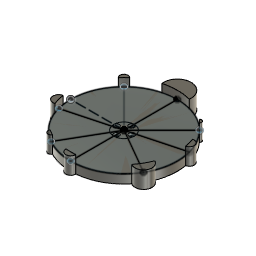
Baseplate_v3 (Autodesk Fusion 360 design; units mm, degrees)
Autodesk Fusion 360 part; units mm, degrees
note: some values were not read from the file. Set by a fixed rule: which face or edge a step refers to.
sketch "Sketch1" plane through (0, 0, 0) normal (0, 0, 1) x (1, 0, 0) in component "Component"
  circle A0 centre (0, 0) radius 60
  circle A1 centre (0, 0) radius 11.5
  dimension "d1" = 120
  dimension "d2" = 23
  constraint coincident A0.centre A1.centre
  measures "d1" diameter of A0
  measures "d2" diameter of A1
extrude "Extrude1" add sketch "Sketch1" along normal blind 5 makes body 1 in component "Component"
sketch "Sketch1 (2)" plane through (0, 0, 5) normal (0, 0, 1) x (-1, 0, 0) in component "Component'"
  circle A0 centre (0, 0) radius 11.5
  circle A1 centre (0, 0) radius 60
  circle A2 centre (0, 0) radius 11.5
  constraint concentric A0 A2
extrude "Extrude1'" add sketch "Sketch1 (2)" along normal blind 2 separate body contours A0 A2 makes body 2 in component "Component'"
move_face "MoveFace1" to x (1, 0, 0) y (0, 1, 0) z (0, 0, 1) at (0, 0, -5) 1 faces at (-11.4857, 0.5732, 6.3333) on bodies 2 in component "Component'"
sketch "Sketch2" plane through (0, 0, 7) normal (0, 0, 1) x (-1, 0, 0) in component "Component'"
  circle A0 centre (0, 0) radius 11.5
sketch "Sketch1 (3)" plane through (0, 0, 7) normal (0, 0, 1) x (-1, 0, 0) in component "Component''"
  circle A0 centre (0, 0) radius 11.5
  circle A1 centre (8.5, 0) radius 1.5
  circle A2 centre (0, -8.5) radius 1.5
  circle A3 centre (-8.5, 0) radius 1.5
  circle A4 centre (0, 8.5) radius 1.5
  dimension "d7" = 23
  dimension "d8" = 3
  dimension "d9" = 3
  dimension "d10" = 3
  dimension "d11" = 3
  measures "d7" diameter of A0
  measures "d8" diameter of A1
  measures "d9" diameter of A2
  measures "d10" diameter of A3
  measures "d11" diameter of A4
extrude "Extrude2" cut sketch "Sketch1 (3)" against normal blind 4.5 contours A1 | A2 | A3 | A4 bodies 2 in component "Component'"
extrude "Extrude2'" add 1 faces at (43.5671, -3.5522, 5) along direction (0, 0, 1) blind 5 on bodies 1 bodies 1 in component "Component"
sketch "Sketch1 (4)" plane through (0, 0, 7) normal (0, 0, 1) x (-1, 0, 0) in component "Component'''"
  circle A0 centre (-8.5, 0) radius 2.5
  circle A1 centre (0, 8.5) radius 2.5
  circle A2 centre (8.5, 0) radius 2.5
  circle A3 centre (0, -8.5) radius 2.5
  dimension "d16" = 5
  dimension "d17" = 5
  dimension "d18" = 5
  dimension "d19" = 5
  measures "d16" diameter of A0
  measures "d17" diameter of A1
  measures "d18" diameter of A2
  measures "d19" diameter of A3
extrude "Extrude3" add sketch "Sketch2" along normal blind 3 bodies 2 in component "Component'"
extrude "Extrude4" cut sketch "Sketch1 (4)" along normal blind 7.5 bodies 2 in component "Component'"
hole "Hole1" at (-8.5, 0, 10) direction (0, 0, -1) diameter 6 depth 3 tip angle 180 bodies 2 in component "Component'"
hole "Hole2" at (0, -8.5, 10) direction (0, 0, -1) diameter 6 depth 3 tip angle 180 bodies 2 in component "Component'"
hole "Hole3" at (8.5, 0, 10) direction (0, 0, -1) diameter 6 depth 3 tip angle 180 bodies 2 in component "Component'"
hole "Hole4" at (0, 8.5, 10) direction (0, 0, -1) diameter 6 depth 3 tip angle 180 bodies 2 in component "Component'"
sketch "Sketch1 (5)" plane through (0, 0, 10) normal (0, 0, 1) x (-1, 0, 0) in component "poles"
  circle A0 centre (0, 0) radius 11.5
  circle A1 centre (0, 0) radius 60
  circle A2 centre (0, 0) radius 60
  line L0 (0, 0) -> (57.9555, 15.5291)
  line L1 (0, 0) -> (60, 0) construction
  line L2 (0, 0) -> (30, 51.9615)
  line L3 (0, 0) -> (60, 0) construction
  line L4 (0, 0) -> (0, 60)
  line L5 (0, 0) -> (-51.9615, 30)
  line L6 (0, 0) -> (-57.9555, -15.5291)
  line L7 (0, 0) -> (60, 0) construction
  line L8 (0, 0) -> (42.4264, -42.4264)
  line L9 (0, 0) -> (60, 0) construction
  line L10 (0, 0) -> (0, -60)
  line L11 (0, 0) -> (-42.4264, -42.4264)
  circle A3 centre (42.4264, -42.4264) radius 2.5
  circle A4 centre (42.4264, -42.4264) radius 2.5
  circle A5 centre (0, -60) radius 2.5
  circle A6 centre (-42.4264, -42.4264) radius 2.5
  circle A7 centre (60, 0) radius 2.5
  circle A8 centre (57.9555, 15.5291) radius 2.5
  circle A9 centre (30, 51.9615) radius 2.5
  circle A10 centre (0, 60) radius 2.5
  circle A11 centre (-51.9615, 30) radius 2.5
  dimension "d36" = 15
  dimension "d37" = 60
  dimension "d38" = 60
  dimension "d39" = 165
  dimension "d40" = 60
  dimension "d41" = 45
  dimension "d42" = 135
  dimension "d43" = 5
  dimension "d44" = 5
  dimension "d45" = 5
  dimension "d46" = 5
  dimension "d47" = 5
  dimension "d48" = 5
  dimension "d49" = 5
  dimension "d50" = 5
  dimension "d51" = 5
  constraint concentric A0 A2
  constraint horizontal L1
  constraint coincident A0.centre A1.centre
  constraint horizontal L3
  constraint vertical L4
  constraint coincident A2 L5.end
  constraint perpendicular L2 L5
  constraint horizontal L7
  constraint horizontal L9
  constraint coincident A2 L10.end
  constraint perpendicular L7 L10
  constraint coincident L8.end A3.centre
  constraint coincident L10.end A5.centre
  constraint coincident L11.end A6.centre
  constraint coincident L1.end L3.end
  constraint coincident L0.end A8.centre
  constraint coincident L2.end A9.centre
  constraint coincident L4.end A10.centre
  constraint coincident L5.end A11.centre
  measures "d36" angle of L0 L1
  measures "d37" angle of L2 L3
  measures "d38" distance of A0.centre L5.end
  measures "d39" angle of L6 L7
  measures "d40" distance of A0.centre L6.end
  measures "d41" angle of L8 L9
  measures "d42" angle of L10 L11
  measures "d43" diameter of A3
  measures "d44" diameter of A4
  measures "d45" diameter of A5
  measures "d46" diameter of A6
  measures "d47" diameter of A7
  measures "d48" diameter of A8
  measures "d49" diameter of A9
  measures "d50" diameter of A10
  measures "d51" diameter of A11
extrude "Extrude1''" add sketch "Sketch1 (5)" along normal blind 9 separate body contours A1 A2 A8 | A1 A2 A3 A4 | A1 A2 A9 | A1 A2 A7 | A1 A2 A5 | A1 A2 A10 | A1 A2 A11 | A1 A2 A6 picked at (60.7968, -0.5156) makes body 3 at (2.0546, 61.4243, 13) makes body 4 at (-2.4929, -60.1889, 16) makes body 5 at (-59.9493, -17.0374, 13) makes body 6 at (40.7077, 44.2419, 16) makes body 7 at (-44.0157, 44.3562, 13) makes body 8 at (-32.4952, -51.8063, 13) makes body 9 at (-60.1889, -2.4929, 13) makes body 10 at (53.8468, -31.6419, 16) in component "poles"
extrude "Extrude2''" add 8 faces at (0, -60.8295, 10) (-30.4147, -52.6799, 10) (-58.7568, -15.7438, 10) (-60.8295, 0, 10) (-43.0129, 43.0129, 10) (43.0129, 43.0129, 10) (52.6799, -30.4147, 10) (0, 60.8295, 10) along direction (0, 0, -1) blind 10 on bodies 3 4 5 6 7 8 9 10 bodies 4 3 5 6 7 8 9 10 in component "poles"
move_body "Move1" bodies 9 to x (-0.965926, -0.258819, 0) y (0.258819, -0.965926, 0) z (0, 0, 1) at (-0.0081, 0.0136, 0) in component "poles"
extrude "Extrude3'" add 2 faces at (0, 60.8295, 19) (-30.4147, -52.6799, 19) along direction (0, 0, -1) blind 4 on bodies 3 8 bodies 3 8 in component "poles"
extrude "Extrude4'" cut 2 faces at (0, -60.8295, 19) (43.0129, 43.0129, 19) along direction (0, 0, 1) blind 6.5 on bodies 4 6 bodies 4 6 in component "poles"
extrude "Extrude5" add 2 faces at (58.7487, 15.7575, 19) (-43.0129, 43.0129, 19) along direction (0, 0, -1) blind 1 on bodies 7 9 bodies 9 7 in component "poles"
move_face "OffsetFaces1" offset 4 2 faces at (-59.9493, -17.0374, 13) (-60.0197, -16.9395, 6.6667) on bodies 5 in component "poles"
move_face "OffsetFaces2" offset 2 3 faces at (-44.0157, 44.3562, 12.6667) (-44.5003, 43.8224, 18.3333) (-44.1069, 44.2773, 3.3333) on bodies 7 in component "poles"
move_face "OffsetFaces3" offset 13 3 faces at (2.0546, 61.4243, 11.6667) (-2.3756, 60.7788, 17.6667) (1.9835, 61.5217, 3.3333) on bodies 3 in component "poles"
move_face "OffsetFaces4" offset 3 3 faces at (57.4847, 17.9996, 12.6667) (58.6604, 13.1466, 18.3333) (57.4847, 17.9996, 3.3333) on bodies 9 in component "poles"
move_face "OffsetFaces5" offset 7 1 faces at (53.7654, -31.7309, 12.6667) on bodies 10 in component "poles"
move_face "OffsetFaces6" offset 3 2 faces at (-2.4929, -60.1889, 16) (-2.4396, -60.5464, 3.3333) on bodies 4 in component "poles"
move_face "OffsetFaces7" offset 1 3 faces at (-32.4952, -51.8063, 11.6667) (-28.3321, -53.8238, 17.6667) (-32.4998, -51.9268, 3.3333) on bodies 8 in component "poles"
component "Component" placed x (1, 0, 0) y (0, 1, 0) z (0, 0, 1) at (0, 0, 0)
component "Component'" placed x (1, 0, 0) y (0, 1, 0) z (0, 0, 1) at (0, 0, 0)
component "Component''" placed x (1, 0, 0) y (0, 1, 0) z (0, 0, 1) at (0, 0, 0)
component "Component'''" placed x (1, 0, 0) y (0, 1, 0) z (0, 0, 1) at (0, 0, 0)
component "poles" placed x (1, 0, 0) y (0, 1, 0) z (0, 0, 1) at (0, 0, 0)
